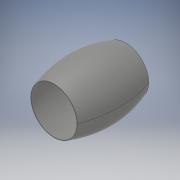
# Autodesk Inventor part: Form
Saved by Autodesk Inventor 2018.3 (Build 223284000, 284)
## iProperties
Created: 2018-07-22
Part Number: Form
Material: Generisch
Document SubType Name: Modeling
Designer: JochenAlt
Density: 1 g/cm^3
Appearance: Textur - grau
Author: JochenAlt
Autodesk Inventor part; units mm, degrees
ref_plane "YZ Plane" through (0, 0, 0) normal (1, 0, 0) x (0, 1, 0)
ref_plane "XZ Plane" through (0, 0, 0) normal (0, 1, 0) x (-1, 0, 0)
ref_plane "XY Plane" through (0, 0, 0) normal (0, 0, 1) x (1, 0, 0)
sketch "Skizze3" plane through (0, 0, 0) normal (0, 0, 1) x (1, 0, 0)
  line L0 (0, 279.6015) -> (0, -256.3881) construction
  line L1 (-136.9115, 0) -> (191.4687, 0) construction
  line L2 (92, 200) -> (90, 200)
  circle A0 centre (0, 0) radius 90 construction
  circle A1 centre (0, -90) radius 89.8182 construction
  line L3 (92, -90) -> (94, -90)
  line L4 (92, -90) -> (142.5573, 65.056) construction
  line L5 (142.5573, 65.056) -> (90, 200) construction
  spline S0 degree 2 poles (92, -90) (142.5573, 65.056) (90, 200) knots 1 1 1 2 2 2
  line L6 (92, 200) -> (144.5573, 65.056) construction
  line L7 (144.5573, 65.056) -> (94, -90) construction
  spline S1 degree 2 poles (92, 200) (144.5573, 65.056) (94, -90) knots 1 1 1 2 2 2
  line L8 (142.5573, 65.056) -> (144.5573, 65.056) construction
  line L9 (142.5573, 65.056) -> (144.5573, 65.056) construction
  point P0 (90, 149.8145)
  dimension "d7" = 200
  dimension "d11" = 2
  dimension "d12" = 92
  dimension "d13" = 180
  dimension "d14" = 90
  dimension "d15" = 90
  dimension "d18" = 2
  dimension "d19" = 2
  constraints: 8 end point, 4 horizontal, 3 coincident, 2 centre point, 2 point on line, 1 parallel, 6 other
  measures "d7" distance between parallel lines of L1 L2
  measures "d11" distance of L2.start L2.end
  measures "d12" distance from line of L0 L3.start
  measures "d13" diameter of A0
  measures "d14" distance of A1.centre point (0, 0)
  measures "d15" distance from line of L0 L2.end
  measures "d18" distance of L3.end L3.start
  measures "d19" distance of L8.start L8.end
revolve "Umdrehung1" add sketch "Skizze3" angle 360 about axis through (0, 0, 0) along (0, -1, 0)
sketch "Skizze6" plane through (0, 0, 0) normal (1, 0, 0) x (0, 1, 0)
  line L0 (-40, 0) -> (240, 0) construction
  line L1 (0, 126) -> (0, -126) construction
  line L2 (179, 25) -> (179, -25)
  line L3 (184, 25) -> (179, 25)
  line L4 (179, -25) -> (184, -25)
  line L5 (184, -25) -> (184, 25)
  line L6 (200, 90) -> (200, -90) projected
  point P0 (0, 0)
  point P1 (200, 0)
  dimension "d35" = 50
  dimension "d49" = 16
  dimension "d51" = 5
  constraints: 8 end point, 2 vertical, 1 horizontal, 1 parallel, 1 other
  measures "d35" distance of L2.start L2.end
  measures "d49" distance between parallel lines of L6 L5
  measures "d51" distance of L2.end L4.end
extrude "Extrusion4" add sketch "Skizze6" along normal up to next separate body
sketch "Skizze7" plane through (0, 0, 0) normal (0, 1, 0) x (-1, 0, 0)
  arc A0 (-91.5453, 13.2558) -> (-91.5453, -13.2558) centre (0, 0) ccw
  circle A1 centre (-80, 0) radius 7.6
  line L0 (-77.5669, -11.2317) -> (-91.5453, -13.2558)
  line L1 (-77.5669, 11.2317) -> (-91.5453, 13.2558)
  line L2 (-92, 0) -> (-118.7883, 0) construction
  line L3 (-69, 1.3349) -> (-69, -1.3349)
  arc A2 (-69, 1.3349) -> (-77.5669, 11.2317) centre (-79, 1.3349) ccw
  arc A3 (-77.5669, -11.2317) -> (-69, -1.3349) centre (-79, -1.3349) ccw
  circle A4 centre (-80, 0) radius 6.6
  line L4 (-91.5453, -13.2558) -> (-130, -18.824)
  line L5 (-91.5453, 13.2558) -> (-130, 18.824)
  line L6 (-130, -18.824) -> (-130, 18.824)
  line L7 (-202.3802, 0) -> (202.3802, 0) construction
  line L8 (-84.6131, 10.2311) -> (-84.3264, 12.2105) construction
  circle A5 centre (0, 0) radius 90 construction
  line L9 (0, 0) -> (-44.9, -77.7691) construction
  line L10 (0, 0) -> (-44.9, 77.7691) construction
  arc A6 (-44.9, 77.7691) -> (-44.9, -77.7691) centre (0, 0) ccw
  arc A7 (-34.9, 60.4486) -> (-34.9, -60.4486) centre (0, 0) ccw
  line L11 (-44.9, -77.7691) -> (-34.9, -60.4486)
  line L12 (-44.9, 77.7691) -> (-34.9, 60.4486)
  point P0 (-69, 9.9912)
  point P1 (-94, 0)
  point P2 (-90, 0)
  dimension "d32" = 185
  dimension "d40" = 15.2
  dimension "d50" = 80
  dimension "d52" = 10
  dimension "d53" = 1
  dimension "d55" = 11
  dimension "d56" = 50
  dimension "d67" = 2
  dimension "d70" = 120
  dimension "d71" = 0.2
  dimension "d72" = 20
  constraints: 22 end point, 10 point on circle, 7 centre point, 7 point on line, 4 coincident, 4 tangent, 2 collinear, 2 vertical, 1 equal radius, 1 horizontal alignment, 1 perpendicular, 2 other
  measures "d32" diameter of A0
  measures "d40" diameter of A1
  measures "d50" distance of A1.centre point (0, 0)
  measures "d52" radius of A2
  measures "d53" radial gap between concentric circles of A4 A1
  measures "d55" distance from line of A1.centre L3
  measures "d56" distance from line of L6 A1.centre
  measures "d67" distance of L8.start L8.end
  measures "d70" angle of L10 L9
  measures "d72" radial gap between concentric circles of A6 A7
extrude "Extrusion5" cut sketch "Skizze7" along normal through all both and the other way through all contours L1 A6 L0 A0 | A0 L4 L6 L5 | L1 A2 A7 A3 L0 A6 | A2 L3 A3 A7 keep common part bodies 2
extrude "Extrusion8" add sketch "Skizze7" along normal blind 1 from surface at 179 contours A1 bodies 2
extrude "Extrusion9" add sketch "Skizze7" along normal blind 1 from surface at 179 contours A1 bodies 2
pattern_circular "Runde Anordnung2" count 3 over 360 about axis through (0, -10, 0) along (0, 1, 0) bodies 2
combine bodies "Kombinieren2" operation type add bodies to combine 2 1
extrude "Extrusion10" add sketch "Skizze7" against normal blind 1 from surface at 200 separate body contours A6 L12 A7 A2 L1 | L1 A2 A7 A3 L0 A6 | L0 A3 A7 L11 A6 | A1
extrude "Extrusion11" add sketch "Skizze7" against normal blind 4 from surface at 199 contours A6 L12 A7 A2 L1 | L1 A2 A7 A3 L0 A6 | L0 A3 A7 L11 A6 bodies 3
pattern_circular "Runde Anordnung3" count 3 over 360 about axis through (0, -10, 0) along (0, 1, 0) of "Extrusion10", "Extrusion11" bodies 3
equation "\"d14\" = 0.5 * d13"
equation "\"d18\" = d17"
equation "\"d16\" = d11"
equation "\"d17\" = d16"
